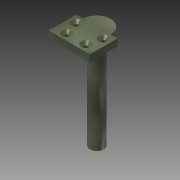
# Autodesk Inventor part: 夹具固定销
Saved by Autodesk Inventor 2015 (Build 190159000, 159)
## iProperties
Created: 2017-05-02
Part Number: 夹具固定销
Material: 常规
Document SubType Name: Modeling
Designer: Administrator
Density: 1 g/cm^3
Appearance: 预制平滑
Author: Administrator
Autodesk Inventor part; units mm, degrees
ref_plane "YZ Plane" through (0, 0, 0) normal (1, 0, 0) x (0, 1, 0)
ref_plane "XZ Plane" through (0, 0, 0) normal (0, 1, 0) x (-1, 0, 0)
ref_plane "XY Plane" through (0, 0, 0) normal (0, 0, 1) x (1, 0, 0)
sketch "草图1" plane through (0, 0, 0) normal (0, 0, 1) x (1, 0, 0)
  arc A0 (10, 0) -> (-10, 0) centre (0, 0) ccw
  line L0 (-15, 0) -> (15, 0)
  line L1 (15, 0) -> (15, -20)
  line L2 (15, -20) -> (-15, -20)
  line L3 (-15, -20) -> (-15, 0)
  circle A1 centre (10, -5) radius 1.5
  circle A2 centre (7, -15) radius 1.5
  circle A3 centre (-10, -5) radius 1.5
  circle A4 centre (-7, -15) radius 1.5
  dimension "d0" = 20
  dimension "d1" = 30
  dimension "d2" = 20
  dimension "d3" = 3
  dimension "d4" = 3
  dimension "d5" = 3
  dimension "d6" = 3
  dimension "d7" = 5
  dimension "d8" = 5
  dimension "d9" = 5
  dimension "d10" = 5
  dimension "d11" = 8
  dimension "d12" = 5
  dimension "d13" = 5
  dimension "d14" = 8
  constraints: 8 end point, 5 centre point, 2 coincident, 2 parallel, 2 point on circle, 2 point on line, 1 horizontal, 1 midpoint, 1 perpendicular
  measures "d0" diameter of A0
  measures "d1" distance of L1.end L2.end
  measures "d2" distance of L0.end L1.end
  measures "d3" diameter of A1
  measures "d4" diameter of A2
  measures "d5" diameter of A3
  measures "d6" diameter of A4
  measures "d7" distance from line of L1 A1.centre
  measures "d8" distance from line of L0 A1.centre
  measures "d9" distance from line of L3 A3.centre
  measures "d10" distance from line of L0 A3.centre
  measures "d11" distance from line of L1 A2.centre
  measures "d12" distance from line of L2 A2.centre
  measures "d13" distance from line of L2 A4.centre
  measures "d14" distance from line of L3 A4.centre
extrude "拉伸1" add sketch "草图1" against normal blind 5
sketch "草图2" plane through (0, 0, -5) normal (0, 0, -1) x (-1, 0, 0)
  circle A0 centre (0, 0) radius 5
  dimension "d17" = 10
  constraints: 1 centre point, 1 coincident
  measures "d17" diameter of A0
extrude "拉伸2" add sketch "草图2" along normal blind 70
chamfer "倒角1" distance 2 angle 45 4 edges at (-11.5, -5, 0) (-8.5, -15, 0) (5.5, -15, 0) (8.5, -5, 0)
